Autodesk Inventor part; units mm, degrees
(part 3 of 7)
  arc A519 (-46.3463, -31.4916) -> (-46.3463, -35.4916) centre (-46.3463, -33.4916) ccw
  arc A520 (-46.3463, -31.4916) -> (-46.3463, -35.4916) centre (-46.3463, -33.4916) ccw
  arc A521 (-46.3463, -31.4916) -> (-46.3463, -35.4916) centre (-46.3463, -33.4916) ccw
  arc A522 (-46.3463, -31.4916) -> (-46.3463, -35.4916) centre (-46.3463, -33.4916) ccw
  arc A523 (-46.3463, -31.4916) -> (-46.3463, -35.4916) centre (-46.3463, -33.4916) ccw
  arc A524 (-52.9119, -35.4916) -> (-52.9119, -31.4916) centre (-52.9119, -33.4916) ccw
  arc A525 (-52.9119, -35.4916) -> (-52.9119, -31.4916) centre (-52.9119, -33.4916) ccw
  arc A526 (-52.9119, -35.4916) -> (-52.9119, -31.4916) centre (-52.9119, -33.4916) ccw
  arc A527 (-52.9119, -35.4916) -> (-52.9119, -31.4916) centre (-52.9119, -33.4916) ccw
  line L460 (-42.4124, -24.5346) -> (-55.8468, -24.5346)
  line L461 (-55.8468, -28.5346) -> (-42.4124, -28.5346)
  line L462 (-55.8468, -28.5346) -> (-42.4124, -28.5346)
  line L463 (-55.8468, -28.5346) -> (-42.4124, -28.5346)
  line L464 (-55.8468, -28.5346) -> (-42.4124, -28.5346)
  line L465 (-55.8468, -28.5346) -> (-42.4124, -28.5346)
  line L466 (-42.4124, -24.5346) -> (-55.8468, -24.5346)
  line L467 (-42.4124, -24.5346) -> (-55.8468, -24.5346)
  line L468 (-42.4124, -24.5346) -> (-55.8468, -24.5346)
  line L469 (-42.4124, -24.5346) -> (-55.8468, -24.5346)
  arc A528 (-86.3463, -31.4916) -> (-86.3463, -35.4916) centre (-86.3463, -33.4916) ccw
  arc A529 (-86.3463, -31.4916) -> (-86.3463, -35.4916) centre (-86.3463, -33.4916) ccw
  arc A530 (-86.3463, -31.4916) -> (-86.3463, -35.4916) centre (-86.3463, -33.4916) ccw
  arc A531 (-92.9119, -35.4916) -> (-92.9119, -31.4916) centre (-92.9119, -33.4916) ccw
  line L470 (-82.4124, -24.5346) -> (-95.8468, -24.5346)
  line L471 (-95.8468, -28.5346) -> (-82.4124, -28.5346)
  line L472 (-86.3463, -35.4916) -> (-72.9119, -35.4916)
  line L473 (-86.3463, -35.4916) -> (-72.9119, -35.4916)
  line L474 (-86.3463, -35.4916) -> (-72.9119, -35.4916)
  line L475 (-72.9119, -31.4916) -> (-86.3463, -31.4916)
  line L476 (-72.9119, -31.4916) -> (-86.3463, -31.4916)
  line L477 (-72.9119, -31.4916) -> (-86.3463, -31.4916)
  arc A532 (-75.8468, -24.5346) -> (-75.8468, -28.5346) centre (-75.8468, -26.5346) ccw
  arc A533 (-75.8468, -24.5346) -> (-75.8468, -28.5346) centre (-75.8468, -26.5346) ccw
  arc A534 (-75.8468, -24.5346) -> (-75.8468, -28.5346) centre (-75.8468, -26.5346) ccw
  arc A535 (-75.8468, -24.5346) -> (-75.8468, -28.5346) centre (-75.8468, -26.5346) ccw
  arc A536 (-82.4124, -28.5346) -> (-82.4124, -24.5346) centre (-82.4124, -26.5346) ccw
  line L478 (-66.3463, -35.4916) -> (-52.9119, -35.4916)
  line L479 (-52.9119, -31.4916) -> (-66.3463, -31.4916)
  line L480 (-52.9119, -31.4916) -> (-66.3463, -31.4916)
  line L481 (-66.3463, -35.4916) -> (-52.9119, -35.4916)
  line L482 (-52.9119, -31.4916) -> (-66.3463, -31.4916)
  line L483 (-52.9119, -31.4916) -> (-66.3463, -31.4916)
  line L484 (-52.9119, -31.4916) -> (-66.3463, -31.4916)
  line L485 (-66.3463, -35.4916) -> (-52.9119, -35.4916)
  line L486 (-66.3463, -35.4916) -> (-52.9119, -35.4916)
  line L487 (-66.3463, -35.4916) -> (-52.9119, -35.4916)
  line L488 (-46.3463, -35.4916) -> (-32.9119, -35.4916)
  line L489 (-32.9119, -31.4916) -> (-46.3463, -31.4916)
  line L490 (-32.9119, -31.4916) -> (-46.3463, -31.4916)
  line L491 (-46.3463, -35.4916) -> (-32.9119, -35.4916)
  line L492 (-32.9119, -31.4916) -> (-46.3463, -31.4916)
  line L493 (-32.9119, -31.4916) -> (-46.3463, -31.4916)
  line L494 (-32.9119, -31.4916) -> (-46.3463, -31.4916)
  line L495 (-46.3463, -35.4916) -> (-32.9119, -35.4916)
  line L496 (-46.3463, -35.4916) -> (-32.9119, -35.4916)
  line L497 (-46.3463, -35.4916) -> (-32.9119, -35.4916)
  line L498 (-46.3463, -35.4916) -> (-32.9119, -35.4916)
  line L499 (-32.9119, -31.4916) -> (-46.3463, -31.4916)
  arc A537 (-55.8468, -24.5346) -> (-55.8468, -28.5346) centre (-55.8468, -26.5346) ccw
  arc A538 (-55.8468, -24.5346) -> (-55.8468, -28.5346) centre (-55.8468, -26.5346) ccw
  arc A539 (-55.8468, -24.5346) -> (-55.8468, -28.5346) centre (-55.8468, -26.5346) ccw
  arc A540 (-62.4124, -28.5346) -> (-62.4124, -24.5346) centre (-62.4124, -26.5346) ccw
  arc A541 (-55.8468, -24.5346) -> (-55.8468, -28.5346) centre (-55.8468, -26.5346) ccw
  arc A542 (-55.8468, -24.5346) -> (-55.8468, -28.5346) centre (-55.8468, -26.5346) ccw
  arc A543 (-55.8468, -24.5346) -> (-55.8468, -28.5346) centre (-55.8468, -26.5346) ccw
  arc A544 (-55.8468, -24.5346) -> (-55.8468, -28.5346) centre (-55.8468, -26.5346) ccw
  arc A545 (-62.4124, -28.5346) -> (-62.4124, -24.5346) centre (-62.4124, -26.5346) ccw
  arc A546 (-62.4124, -28.5346) -> (-62.4124, -24.5346) centre (-62.4124, -26.5346) ccw
  arc A547 (-66.3463, -31.4916) -> (-66.3463, -35.4916) centre (-66.3463, -33.4916) ccw
  arc A548 (-72.9119, -35.4916) -> (-72.9119, -31.4916) centre (-72.9119, -33.4916) ccw
  arc A549 (-66.3463, -31.4916) -> (-66.3463, -35.4916) centre (-66.3463, -33.4916) ccw
  line L500 (-62.4124, -24.5346) -> (-75.8468, -24.5346)
  line L501 (-75.8468, -28.5346) -> (-62.4124, -28.5346)
  arc A550 (-72.9119, -35.4916) -> (-72.9119, -31.4916) centre (-72.9119, -33.4916) ccw
  line L502 (-62.4124, -24.5346) -> (-75.8468, -24.5346)
  line L503 (-75.8468, -28.5346) -> (-62.4124, -28.5346)
  arc A551 (-66.3463, -31.4916) -> (-66.3463, -35.4916) centre (-66.3463, -33.4916) ccw
  arc A552 (-66.3463, -31.4916) -> (-66.3463, -35.4916) centre (-66.3463, -33.4916) ccw
  arc A553 (-66.3463, -31.4916) -> (-66.3463, -35.4916) centre (-66.3463, -33.4916) ccw
  line L504 (-62.4124, -24.5346) -> (-75.8468, -24.5346)
  line L505 (-75.8468, -28.5346) -> (-62.4124, -28.5346)
  arc A554 (-72.9119, -35.4916) -> (-72.9119, -31.4916) centre (-72.9119, -33.4916) ccw
  arc A555 (-106.3463, -31.4916) -> (-106.3463, -35.4916) centre (-106.3463, -33.4916) ccw
  arc A556 (-95.8468, -24.5346) -> (-95.8468, -28.5346) centre (-95.8468, -26.5346) ccw
  line L506 (-92.9119, -31.4916) -> (-106.3463, -31.4916)
  line L507 (-106.3463, -35.4916) -> (-92.9119, -35.4916)
  arc A557 (-35.8468, -24.5346) -> (-35.8468, -28.5346) centre (-35.8468, -26.5346) ccw
  arc A558 (-35.8468, -24.5346) -> (-35.8468, -28.5346) centre (-35.8468, -26.5346) ccw
  arc A559 (-35.8468, -24.5346) -> (-35.8468, -28.5346) centre (-35.8468, -26.5346) ccw
  arc A560 (-42.4124, -28.5346) -> (-42.4124, -24.5346) centre (-42.4124, -26.5346) ccw
  arc A561 (-42.4124, -28.5346) -> (-42.4124, -24.5346) centre (-42.4124, -26.5346) ccw
  arc A562 (-35.8468, -24.5346) -> (-35.8468, -28.5346) centre (-35.8468, -26.5346) ccw
  arc A563 (-35.8468, -24.5346) -> (-35.8468, -28.5346) centre (-35.8468, -26.5346) ccw
  arc A564 (-35.8468, -24.5346) -> (-35.8468, -28.5346) centre (-35.8468, -26.5346) ccw
  arc A565 (-35.8468, -24.5346) -> (-35.8468, -28.5346) centre (-35.8468, -26.5346) ccw
  arc A566 (-35.8468, -24.5346) -> (-35.8468, -28.5346) centre (-35.8468, -26.5346) ccw
  arc A567 (-35.8468, -24.5346) -> (-35.8468, -28.5346) centre (-35.8468, -26.5346) ccw
  arc A568 (-42.4124, -28.5346) -> (-42.4124, -24.5346) centre (-42.4124, -26.5346) ccw
  arc A569 (-42.4124, -28.5346) -> (-42.4124, -24.5346) centre (-42.4124, -26.5346) ccw
  arc A570 (-42.4124, -28.5346) -> (-42.4124, -24.5346) centre (-42.4124, -26.5346) ccw
  arc A571 (44.1532, -10.5346) -> (44.1532, -14.5346) centre (44.1532, -12.5346) ccw
  arc A572 (44.1532, -10.5346) -> (44.1532, -14.5346) centre (44.1532, -12.5346) ccw
  arc A573 (44.1532, -10.5346) -> (44.1532, -14.5346) centre (44.1532, -12.5346) ccw
  arc A574 (44.1532, -10.5346) -> (44.1532, -14.5346) centre (44.1532, -12.5346) ccw
  arc A575 (44.1532, -10.5346) -> (44.1532, -14.5346) centre (44.1532, -12.5346) ccw
  arc A576 (44.1532, -10.5346) -> (44.1532, -14.5346) centre (44.1532, -12.5346) ccw
  arc A577 (44.1532, -10.5346) -> (44.1532, -14.5346) centre (44.1532, -12.5346) ccw
  arc A578 (33.6537, -17.4916) -> (33.6537, -21.4916) centre (33.6537, -19.4916) ccw
  arc A579 (27.0881, -21.4916) -> (27.0881, -17.4916) centre (27.0881, -19.4916) ccw
  arc A580 (27.0881, -21.4916) -> (27.0881, -17.4916) centre (27.0881, -19.4916) ccw
  arc A581 (33.6537, -17.4916) -> (33.6537, -21.4916) centre (33.6537, -19.4916) ccw
  arc A582 (27.0881, -21.4916) -> (27.0881, -17.4916) centre (27.0881, -19.4916) ccw
  arc A583 (27.0881, -21.4916) -> (27.0881, -17.4916) centre (27.0881, -19.4916) ccw
  arc A584 (27.0881, -21.4916) -> (27.0881, -17.4916) centre (27.0881, -19.4916) ccw
  arc A585 (27.0881, -21.4916) -> (27.0881, -17.4916) centre (27.0881, -19.4916) ccw
  arc A586 (33.6537, -17.4916) -> (33.6537, -21.4916) centre (33.6537, -19.4916) ccw
  arc A587 (33.6537, -17.4916) -> (33.6537, -21.4916) centre (33.6537, -19.4916) ccw
  arc A588 (33.6537, -17.4916) -> (33.6537, -21.4916) centre (33.6537, -19.4916) ccw
  line L508 (24.1532, -14.5346) -> (37.5876, -14.5346)
  line L509 (37.5876, -10.5346) -> (24.1532, -10.5346)
  line L510 (24.1532, -14.5346) -> (37.5876, -14.5346)
  line L511 (24.1532, -14.5346) -> (37.5876, -14.5346)
  line L512 (24.1532, -14.5346) -> (37.5876, -14.5346)
  line L513 (24.1532, -14.5346) -> (37.5876, -14.5346)
  line L514 (24.1532, -14.5346) -> (37.5876, -14.5346)
  line L515 (37.5876, -10.5346) -> (24.1532, -10.5346)
  line L516 (37.5876, -10.5346) -> (24.1532, -10.5346)
  line L517 (37.5876, -10.5346) -> (24.1532, -10.5346)
  line L518 (37.5876, -10.5346) -> (24.1532, -10.5346)
  line L519 (37.5876, -10.5346) -> (24.1532, -10.5346)
  arc A589 (37.5876, -14.5346) -> (37.5876, -10.5346) centre (37.5876, -12.5346) ccw
  arc A590 (37.5876, -14.5346) -> (37.5876, -10.5346) centre (37.5876, -12.5346) ccw
  arc A591 (37.5876, -14.5346) -> (37.5876, -10.5346) centre (37.5876, -12.5346) ccw
  arc A592 (37.5876, -14.5346) -> (37.5876, -10.5346) centre (37.5876, -12.5346) ccw
  arc A593 (37.5876, -14.5346) -> (37.5876, -10.5346) centre (37.5876, -12.5346) ccw
  arc A594 (37.5876, -14.5346) -> (37.5876, -10.5346) centre (37.5876, -12.5346) ccw
  arc A595 (44.1532, -10.5346) -> (44.1532, -14.5346) centre (44.1532, -12.5346) ccw
  arc A596 (47.0881, -21.4916) -> (47.0881, -17.4916) centre (47.0881, -19.4916) ccw
  arc A597 (47.0881, -21.4916) -> (47.0881, -17.4916) centre (47.0881, -19.4916) ccw
  arc A598 (53.6537, -17.4916) -> (53.6537, -21.4916) centre (53.6537, -19.4916) ccw
  arc A599 (47.0881, -21.4916) -> (47.0881, -17.4916) centre (47.0881, -19.4916) ccw
  arc A600 (47.0881, -21.4916) -> (47.0881, -17.4916) centre (47.0881, -19.4916) ccw
  arc A601 (47.0881, -21.4916) -> (47.0881, -17.4916) centre (47.0881, -19.4916) ccw
  arc A602 (53.6537, -17.4916) -> (53.6537, -21.4916) centre (53.6537, -19.4916) ccw
  arc A603 (53.6537, -17.4916) -> (53.6537, -21.4916) centre (53.6537, -19.4916) ccw
  line L520 (57.5876, -10.5346) -> (44.1532, -10.5346)
  line L521 (44.1532, -14.5346) -> (57.5876, -14.5346)
  line L522 (57.5876, -10.5346) -> (44.1532, -10.5346)
  line L523 (44.1532, -14.5346) -> (57.5876, -14.5346)
  line L524 (44.1532, -14.5346) -> (57.5876, -14.5346)
  line L525 (44.1532, -14.5346) -> (57.5876, -14.5346)
  line L526 (44.1532, -14.5346) -> (57.5876, -14.5346)
  line L527 (57.5876, -10.5346) -> (44.1532, -10.5346)
  line L528 (57.5876, -10.5346) -> (44.1532, -10.5346)
  line L529 (57.5876, -10.5346) -> (44.1532, -10.5346)
  arc A604 (57.5876, -14.5346) -> (57.5876, -10.5346) centre (57.5876, -12.5346) ccw
  arc A605 (64.1532, -10.5346) -> (64.1532, -14.5346) centre (64.1532, -12.5346) ccw
  line L530 (53.6537, -21.4916) -> (67.0881, -21.4916)
  line L531 (53.6537, -21.4916) -> (67.0881, -21.4916)
  line L532 (53.6537, -21.4916) -> (67.0881, -21.4916)
  line L533 (67.0881, -17.4916) -> (53.6537, -17.4916)
  line L534 (67.0881, -17.4916) -> (53.6537, -17.4916)
  line L535 (67.0881, -17.4916) -> (53.6537, -17.4916)
  arc A606 (64.1532, -10.5346) -> (64.1532, -14.5346) centre (64.1532, -12.5346) ccw
  arc A607 (64.1532, -10.5346) -> (64.1532, -14.5346) centre (64.1532, -12.5346) ccw
  arc A608 (64.1532, -10.5346) -> (64.1532, -14.5346) centre (64.1532, -12.5346) ccw
  arc A609 (64.1532, -10.5346) -> (64.1532, -14.5346) centre (64.1532, -12.5346) ccw
  arc A610 (57.5876, -14.5346) -> (57.5876, -10.5346) centre (57.5876, -12.5346) ccw
  arc A611 (57.5876, -14.5346) -> (57.5876, -10.5346) centre (57.5876, -12.5346) ccw
  arc A612 (57.5876, -14.5346) -> (57.5876, -10.5346) centre (57.5876, -12.5346) ccw
  arc A613 (57.5876, -14.5346) -> (57.5876, -10.5346) centre (57.5876, -12.5346) ccw
  arc A614 (67.0881, -21.4916) -> (67.0881, -17.4916) centre (67.0881, -19.4916) ccw
  arc A615 (67.0881, -21.4916) -> (67.0881, -17.4916) centre (67.0881, -19.4916) ccw
  arc A616 (67.0881, -21.4916) -> (67.0881, -17.4916) centre (67.0881, -19.4916) ccw
  line L536 (77.5876, -10.5346) -> (64.1532, -10.5346)
  line L537 (77.5876, -10.5346) -> (64.1532, -10.5346)
  line L538 (77.5876, -10.5346) -> (64.1532, -10.5346)
  line L539 (64.1532, -14.5346) -> (77.5876, -14.5346)
  line L540 (64.1532, -14.5346) -> (77.5876, -14.5346)
  line L541 (64.1532, -14.5346) -> (77.5876, -14.5346)
  arc A617 (73.6537, -17.4916) -> (73.6537, -21.4916) centre (73.6537, -19.4916) ccw
  arc A618 (77.5876, -14.5346) -> (77.5876, -10.5346) centre (77.5876, -12.5346) ccw
  arc A619 (77.5876, -14.5346) -> (77.5876, -10.5346) centre (77.5876, -12.5346) ccw
  arc A620 (77.5876, -14.5346) -> (77.5876, -10.5346) centre (77.5876, -12.5346) ccw
  arc A621 (84.1532, -10.5346) -> (84.1532, -14.5346) centre (84.1532, -12.5346) ccw
  arc A622 (84.1532, -10.5346) -> (84.1532, -14.5346) centre (84.1532, -12.5346) ccw
  line L542 (87.0881, -17.4916) -> (73.6537, -17.4916)
  arc A623 (87.0881, -21.4916) -> (87.0881, -17.4916) centre (87.0881, -19.4916) ccw
  line L543 (73.6537, -21.4916) -> (87.0881, -21.4916)
  line L544 (84.1532, -14.5346) -> (97.5876, -14.5346)
  line L545 (97.5876, -10.5346) -> (84.1532, -10.5346)
  arc A624 (97.5876, -14.5346) -> (97.5876, -10.5346) centre (97.5876, -12.5346) ccw
  line L546 (33.6537, -21.4916) -> (47.0881, -21.4916)
  line L547 (47.0881, -17.4916) -> (33.6537, -17.4916)
  line L548 (33.6537, -21.4916) -> (47.0881, -21.4916)
  line L549 (47.0881, -17.4916) -> (33.6537, -17.4916)
  line L550 (47.0881, -17.4916) -> (33.6537, -17.4916)
  line L551 (47.0881, -17.4916) -> (33.6537, -17.4916)
  line L552 (47.0881, -17.4916) -> (33.6537, -17.4916)
  line L553 (33.6537, -21.4916) -> (47.0881, -21.4916)
  line L554 (33.6537, -21.4916) -> (47.0881, -21.4916)
  line L555 (33.6537, -21.4916) -> (47.0881, -21.4916)
  arc A625 (13.6537, -17.4916) -> (13.6537, -21.4916) centre (13.6537, -19.4916) ccw
  arc A626 (13.6537, -17.4916) -> (13.6537, -21.4916) centre (13.6537, -19.4916) ccw
  arc A627 (13.6537, -17.4916) -> (13.6537, -21.4916) centre (13.6537, -19.4916) ccw
  arc A628 (13.6537, -17.4916) -> (13.6537, -21.4916) centre (13.6537, -19.4916) ccw
  arc A629 (13.6537, -17.4916) -> (13.6537, -21.4916) centre (13.6537, -19.4916) ccw
  arc A630 (13.6537, -17.4916) -> (13.6537, -21.4916) centre (13.6537, -19.4916) ccw
  arc A631 (7.0881, -21.4916) -> (7.0881, -17.4916) centre (7.0881, -19.4916) ccw
  arc A632 (7.0881, -21.4916) -> (7.0881, -17.4916) centre (7.0881, -19.4916) ccw
  arc A633 (7.0881, -21.4916) -> (7.0881, -17.4916) centre (7.0881, -19.4916) ccw
  arc A634 (7.0881, -21.4916) -> (7.0881, -17.4916) centre (7.0881, -19.4916) ccw
  arc A635 (17.5876, -14.5346) -> (17.5876, -10.5346) centre (17.5876, -12.5346) ccw
  arc A636 (17.5876, -14.5346) -> (17.5876, -10.5346) centre (17.5876, -12.5346) ccw
  arc A637 (17.5876, -14.5346) -> (17.5876, -10.5346) centre (17.5876, -12.5346) ccw
  arc A638 (17.5876, -14.5346) -> (17.5876, -10.5346) centre (17.5876, -12.5346) ccw
  arc A639 (17.5876, -14.5346) -> (17.5876, -10.5346) centre (17.5876, -12.5346) ccw
  arc A640 (17.5876, -14.5346) -> (17.5876, -10.5346) centre (17.5876, -12.5346) ccw
  arc A641 (24.1532, -10.5346) -> (24.1532, -14.5346) centre (24.1532, -12.5346) ccw
  arc A642 (24.1532, -10.5346) -> (24.1532, -14.5346) centre (24.1532, -12.5346) ccw
  arc A643 (24.1532, -10.5346) -> (24.1532, -14.5346) centre (24.1532, -12.5346) ccw
  arc A644 (24.1532, -10.5346) -> (24.1532, -14.5346) centre (24.1532, -12.5346) ccw
  arc A645 (24.1532, -10.5346) -> (24.1532, -14.5346) centre (24.1532, -12.5346) ccw
  arc A646 (24.1532, -10.5346) -> (24.1532, -14.5346) centre (24.1532, -12.5346) ccw
  arc A647 (24.1532, -10.5346) -> (24.1532, -14.5346) centre (24.1532, -12.5346) ccw
  arc A648 (24.1532, -10.5346) -> (24.1532, -14.5346) centre (24.1532, -12.5346) ccw
  arc A649 (24.1532, -10.5346) -> (24.1532, -14.5346) centre (24.1532, -12.5346) ccw
  arc A650 (4.1532, -10.5346) -> (4.1532, -14.5346) centre (4.1532, -12.5346) ccw
  arc A651 (4.1532, -10.5346) -> (4.1532, -14.5346) centre (4.1532, -12.5346) ccw
  arc A652 (4.1532, -10.5346) -> (4.1532, -14.5346) centre (4.1532, -12.5346) ccw
  arc A653 (4.1532, -10.5346) -> (4.1532, -14.5346) centre (4.1532, -12.5346) ccw
  arc A654 (4.1532, -10.5346) -> (4.1532, -14.5346) centre (4.1532, -12.5346) ccw
  arc A655 (4.1532, -10.5346) -> (4.1532, -14.5346) centre (4.1532, -12.5346) ccw
  arc A656 (4.1532, -10.5346) -> (4.1532, -14.5346) centre (4.1532, -12.5346) ccw
  arc A657 (4.1532, -10.5346) -> (4.1532, -14.5346) centre (4.1532, -12.5346) ccw
  arc A658 (4.1532, -10.5346) -> (4.1532, -14.5346) centre (4.1532, -12.5346) ccw
  arc A659 (-2.4124, -14.5346) -> (-2.4124, -10.5346) centre (-2.4124, -12.5346) ccw
  arc A660 (-2.4124, -14.5346) -> (-2.4124, -10.5346) centre (-2.4124, -12.5346) ccw
  arc A661 (-2.4124, -14.5346) -> (-2.4124, -10.5346) centre (-2.4124, -12.5346) ccw
  arc A662 (-2.4124, -14.5346) -> (-2.4124, -10.5346) centre (-2.4124, -12.5346) ccw
  arc A663 (-32.9119, -21.4916) -> (-32.9119, -17.4916) centre (-32.9119, -19.4916) ccw
  arc A664 (-32.9119, -21.4916) -> (-32.9119, -17.4916) centre (-32.9119, -19.4916) ccw
  arc A665 (-32.9119, -21.4916) -> (-32.9119, -17.4916) centre (-32.9119, -19.4916) ccw
  arc A666 (-32.9119, -21.4916) -> (-32.9119, -17.4916) centre (-32.9119, -19.4916) ccw
  arc A667 (-32.9119, -21.4916) -> (-32.9119, -17.4916) centre (-32.9119, -19.4916) ccw
  arc A668 (-32.9119, -21.4916) -> (-32.9119, -17.4916) centre (-32.9119, -19.4916) ccw
  line L556 (27.0881, -17.4916) -> (13.6537, -17.4916)
  line L557 (13.6537, -21.4916) -> (27.0881, -21.4916)
  line L558 (27.0881, -17.4916) -> (13.6537, -17.4916)
  line L559 (13.6537, -21.4916) -> (27.0881, -21.4916)
  line L560 (13.6537, -21.4916) -> (27.0881, -21.4916)
  line L561 (27.0881, -17.4916) -> (13.6537, -17.4916)
  line L562 (27.0881, -17.4916) -> (13.6537, -17.4916)
  line L563 (27.0881, -17.4916) -> (13.6537, -17.4916)
  line L564 (13.6537, -21.4916) -> (27.0881, -21.4916)
  line L565 (13.6537, -21.4916) -> (27.0881, -21.4916)
  line L566 (13.6537, -21.4916) -> (27.0881, -21.4916)
  line L567 (27.0881, -17.4916) -> (13.6537, -17.4916)
  line L568 (4.1532, -14.5346) -> (17.5876, -14.5346)
  line L569 (4.1532, -14.5346) -> (17.5876, -14.5346)
  line L570 (4.1532, -14.5346) -> (17.5876, -14.5346)
  line L571 (4.1532, -14.5346) -> (17.5876, -14.5346)
  line L572 (4.1532, -14.5346) -> (17.5876, -14.5346)
  line L573 (4.1532, -14.5346) -> (17.5876, -14.5346)
  line L574 (17.5876, -10.5346) -> (4.1532, -10.5346)
  line L575 (17.5876, -10.5346) -> (4.1532, -10.5346)
  line L576 (17.5876, -10.5346) -> (4.1532, -10.5346)
  line L577 (17.5876, -10.5346) -> (4.1532, -10.5346)
  line L578 (17.5876, -10.5346) -> (4.1532, -10.5346)
  line L579 (17.5876, -10.5346) -> (4.1532, -10.5346)
  arc A669 (7.0881, -21.4916) -> (7.0881, -17.4916) centre (7.0881, -19.4916) ccw
  arc A670 (7.0881, -21.4916) -> (7.0881, -17.4916) centre (7.0881, -19.4916) ccw
  line L580 (-6.3463, -21.4916) -> (7.0881, -21.4916)
  line L581 (7.0881, -17.4916) -> (-6.3463, -17.4916)
  line L582 (7.0881, -17.4916) -> (-6.3463, -17.4916)
  line L583 (-6.3463, -21.4916) -> (7.0881, -21.4916)
  line L584 (-6.3463, -21.4916) -> (7.0881, -21.4916)
  line L585 (7.0881, -17.4916) -> (-6.3463, -17.4916)
  line L586 (7.0881, -17.4916) -> (-6.3463, -17.4916)
  line L587 (7.0881, -17.4916) -> (-6.3463, -17.4916)
  line L588 (-6.3463, -21.4916) -> (7.0881, -21.4916)
  line L589 (-6.3463, -21.4916) -> (7.0881, -21.4916)
  line L590 (-6.3463, -21.4916) -> (7.0881, -21.4916)
  line L591 (7.0881, -17.4916) -> (-6.3463, -17.4916)
  arc A671 (-6.3463, -17.4916) -> (-6.3463, -21.4916) centre (-6.3463, -19.4916) ccw
  arc A672 (-6.3463, -17.4916) -> (-6.3463, -21.4916) centre (-6.3463, -19.4916) ccw
  arc A673 (-6.3463, -17.4916) -> (-6.3463, -21.4916) centre (-6.3463, -19.4916) ccw
  arc A674 (-6.3463, -17.4916) -> (-6.3463, -21.4916) centre (-6.3463, -19.4916) ccw
  arc A675 (-6.3463, -17.4916) -> (-6.3463, -21.4916) centre (-6.3463, -19.4916) ccw
  arc A676 (-6.3463, -17.4916) -> (-6.3463, -21.4916) centre (-6.3463, -19.4916) ccw
  arc A677 (-12.9119, -21.4916) -> (-12.9119, -17.4916) centre (-12.9119, -19.4916) ccw
  arc A678 (-12.9119, -21.4916) -> (-12.9119, -17.4916) centre (-12.9119, -19.4916) ccw
  arc A679 (-12.9119, -21.4916) -> (-12.9119, -17.4916) centre (-12.9119, -19.4916) ccw
  arc A680 (-12.9119, -21.4916) -> (-12.9119, -17.4916) centre (-12.9119, -19.4916) ccw
  arc A681 (-12.9119, -21.4916) -> (-12.9119, -17.4916) centre (-12.9119, -19.4916) ccw
  line L592 (-2.4124, -10.5346) -> (-15.8468, -10.5346)
  line L593 (-15.8468, -14.5346) -> (-2.4124, -14.5346)
  line L594 (-2.4124, -10.5346) -> (-15.8468, -10.5346)
  line L595 (-15.8468, -14.5346) -> (-2.4124, -14.5346)
  line L596 (-2.4124, -10.5346) -> (-15.8468, -10.5346)
  line L597 (-15.8468, -14.5346) -> (-2.4124, -14.5346)
  line L598 (-2.4124, -10.5346) -> (-15.8468, -10.5346)
  line L599 (-15.8468, -14.5346) -> (-2.4124, -14.5346)
  line L600 (-2.4124, -10.5346) -> (-15.8468, -10.5346)
  line L601 (-15.8468, -14.5346) -> (-2.4124, -14.5346)
  line L602 (-15.8468, -14.5346) -> (-2.4124, -14.5346)
  line L603 (-2.4124, -10.5346) -> (-15.8468, -10.5346)
  arc A682 (-2.4124, -14.5346) -> (-2.4124, -10.5346) centre (-2.4124, -12.5346) ccw
  arc A683 (-2.4124, -14.5346) -> (-2.4124, -10.5346) centre (-2.4124, -12.5346) ccw
  arc A684 (-15.8468, -10.5346) -> (-15.8468, -14.5346) centre (-15.8468, -12.5346) ccw
  arc A685 (-15.8468, -10.5346) -> (-15.8468, -14.5346) centre (-15.8468, -12.5346) ccw
  arc A686 (-15.8468, -10.5346) -> (-15.8468, -14.5346) centre (-15.8468, -12.5346) ccw
  arc A687 (-15.8468, -10.5346) -> (-15.8468, -14.5346) centre (-15.8468, -12.5346) ccw
  arc A688 (-15.8468, -10.5346) -> (-15.8468, -14.5346) centre (-15.8468, -12.5346) ccw
  arc A689 (-22.4124, -14.5346) -> (-22.4124, -10.5346) centre (-22.4124, -12.5346) ccw
  arc A690 (-22.4124, -14.5346) -> (-22.4124, -10.5346) centre (-22.4124, -12.5346) ccw
  arc A691 (-15.8468, -10.5346) -> (-15.8468, -14.5346) centre (-15.8468, -12.5346) ccw
  arc A692 (-15.8468, -10.5346) -> (-15.8468, -14.5346) centre (-15.8468, -12.5346) ccw
  arc A693 (-22.4124, -14.5346) -> (-22.4124, -10.5346) centre (-22.4124, -12.5346) ccw
  arc A694 (-15.8468, -10.5346) -> (-15.8468, -14.5346) centre (-15.8468, -12.5346) ccw
  arc A695 (-15.8468, -10.5346) -> (-15.8468, -14.5346) centre (-15.8468, -12.5346) ccw
  arc A696 (-22.4124, -14.5346) -> (-22.4124, -10.5346) centre (-22.4124, -12.5346) ccw
  arc A697 (-22.4124, -14.5346) -> (-22.4124, -10.5346) centre (-22.4124, -12.5346) ccw
  arc A698 (-22.4124, -14.5346) -> (-22.4124, -10.5346) centre (-22.4124, -12.5346) ccw
  arc A699 (-26.3463, -17.4916) -> (-26.3463, -21.4916) centre (-26.3463, -19.4916) ccw
  arc A700 (-26.3463, -17.4916) -> (-26.3463, -21.4916) centre (-26.3463, -19.4916) ccw
  arc A701 (-26.3463, -17.4916) -> (-26.3463, -21.4916) centre (-26.3463, -19.4916) ccw
  arc A702 (-26.3463, -17.4916) -> (-26.3463, -21.4916) centre (-26.3463, -19.4916) ccw
  arc A703 (-26.3463, -17.4916) -> (-26.3463, -21.4916) centre (-26.3463, -19.4916) ccw
  arc A704 (-26.3463, -17.4916) -> (-26.3463, -21.4916) centre (-26.3463, -19.4916) ccw
  line L604 (-35.8468, -14.5346) -> (-22.4124, -14.5346)
  line L605 (-35.8468, -14.5346) -> (-22.4124, -14.5346)
  line L606 (-35.8468, -14.5346) -> (-22.4124, -14.5346)
  line L607 (-35.8468, -14.5346) -> (-22.4124, -14.5346)
  line L608 (-35.8468, -14.5346) -> (-22.4124, -14.5346)
  line L609 (-35.8468, -14.5346) -> (-22.4124, -14.5346)
  line L610 (-22.4124, -10.5346) -> (-35.8468, -10.5346)
  line L611 (-22.4124, -10.5346) -> (-35.8468, -10.5346)
  line L612 (-22.4124, -10.5346) -> (-35.8468, -10.5346)
  line L613 (-22.4124, -10.5346) -> (-35.8468, -10.5346)
  line L614 (-22.4124, -10.5346) -> (-35.8468, -10.5346)
  line L615 (-22.4124, -10.5346) -> (-35.8468, -10.5346)
  line L616 (-26.3463, -21.4916) -> (-12.9119, -21.4916)
  line L617 (-12.9119, -17.4916) -> (-26.3463, -17.4916)
  line L618 (-12.9119, -17.4916) -> (-26.3463, -17.4916)
  line L619 (-26.3463, -21.4916) -> (-12.9119, -21.4916)
  line L620 (-12.9119, -17.4916) -> (-26.3463, -17.4916)
  line L621 (-12.9119, -17.4916) -> (-26.3463, -17.4916)
  line L622 (-26.3463, -21.4916) -> (-12.9119, -21.4916)
  line L623 (-12.9119, -17.4916) -> (-26.3463, -17.4916)
  line L624 (-12.9119, -17.4916) -> (-26.3463, -17.4916)
  line L625 (-26.3463, -21.4916) -> (-12.9119, -21.4916)
  line L626 (-26.3463, -21.4916) -> (-12.9119, -21.4916)
  line L627 (-26.3463, -21.4916) -> (-12.9119, -21.4916)
  arc A705 (-12.9119, -21.4916) -> (-12.9119, -17.4916) centre (-12.9119, -19.4916) ccw
  arc A706 (-46.3463, -17.4916) -> (-46.3463, -21.4916) centre (-46.3463, -19.4916) ccw
  arc A707 (-52.9119, -21.4916) -> (-52.9119, -17.4916) centre (-52.9119, -19.4916) ccw
  arc A708 (-46.3463, -17.4916) -> (-46.3463, -21.4916) centre (-46.3463, -19.4916) ccw
  arc A709 (-46.3463, -17.4916) -> (-46.3463, -21.4916) centre (-46.3463, -19.4916) ccw
  arc A710 (-46.3463, -17.4916) -> (-46.3463, -21.4916) centre (-46.3463, -19.4916) ccw
  arc A711 (-46.3463, -17.4916) -> (-46.3463, -21.4916) centre (-46.3463, -19.4916) ccw
  arc A712 (-46.3463, -17.4916) -> (-46.3463, -21.4916) centre (-46.3463, -19.4916) ccw
  arc A713 (-52.9119, -21.4916) -> (-52.9119, -17.4916) centre (-52.9119, -19.4916) ccw
  arc A714 (-52.9119, -21.4916) -> (-52.9119, -17.4916) centre (-52.9119, -19.4916) ccw
  arc A715 (-52.9119, -21.4916) -> (-52.9119, -17.4916) centre (-52.9119, -19.4916) ccw
  arc A716 (-52.9119, -21.4916) -> (-52.9119, -17.4916) centre (-52.9119, -19.4916) ccw
  line L628 (-42.4124, -10.5346) -> (-55.8468, -10.5346)
  line L629 (-55.8468, -14.5346) -> (-42.4124, -14.5346)
  line L630 (-55.8468, -14.5346) -> (-42.4124, -14.5346)
  line L631 (-55.8468, -14.5346) -> (-42.4124, -14.5346)
  line L632 (-55.8468, -14.5346) -> (-42.4124, -14.5346)
  line L633 (-55.8468, -14.5346) -> (-42.4124, -14.5346)
  line L634 (-42.4124, -10.5346) -> (-55.8468, -10.5346)
  line L635 (-42.4124, -10.5346) -> (-55.8468, -10.5346)
  line L636 (-42.4124, -10.5346) -> (-55.8468, -10.5346)
  line L637 (-42.4124, -10.5346) -> (-55.8468, -10.5346)
  arc A717 (-86.3463, -17.4916) -> (-86.3463, -21.4916) centre (-86.3463, -19.4916) ccw
  arc A718 (-86.3463, -17.4916) -> (-86.3463, -21.4916) centre (-86.3463, -19.4916) ccw
  arc A719 (-86.3463, -17.4916) -> (-86.3463, -21.4916) centre (-86.3463, -19.4916) ccw
  arc A720 (-92.9119, -21.4916) -> (-92.9119, -17.4916) centre (-92.9119, -19.4916) ccw
  line L638 (-82.4124, -10.5346) -> (-95.8468, -10.5346)
  line L639 (-95.8468, -14.5346) -> (-82.4124, -14.5346)
  line L640 (-86.3463, -21.4916) -> (-72.9119, -21.4916)
  line L641 (-86.3463, -21.4916) -> (-72.9119, -21.4916)
  line L642 (-86.3463, -21.4916) -> (-72.9119, -21.4916)
  line L643 (-72.9119, -17.4916) -> (-86.3463, -17.4916)
  line L644 (-72.9119, -17.4916) -> (-86.3463, -17.4916)
  line L645 (-72.9119, -17.4916) -> (-86.3463, -17.4916)
  arc A721 (-75.8468, -10.5346) -> (-75.8468, -14.5346) centre (-75.8468, -12.5346) ccw
  arc A722 (-75.8468, -10.5346) -> (-75.8468, -14.5346) centre (-75.8468, -12.5346) ccw
  arc A723 (-75.8468, -10.5346) -> (-75.8468, -14.5346) centre (-75.8468, -12.5346) ccw
  arc A724 (-75.8468, -10.5346) -> (-75.8468, -14.5346) centre (-75.8468, -12.5346) ccw
  arc A725 (-82.4124, -14.5346) -> (-82.4124, -10.5346) centre (-82.4124, -12.5346) ccw
  line L646 (-66.3463, -21.4916) -> (-52.9119, -21.4916)
  line L647 (-52.9119, -17.4916) -> (-66.3463, -17.4916)
  line L648 (-52.9119, -17.4916) -> (-66.3463, -17.4916)
  line L649 (-66.3463, -21.4916) -> (-52.9119, -21.4916)
  line L650 (-52.9119, -17.4916) -> (-66.3463, -17.4916)
  line L651 (-52.9119, -17.4916) -> (-66.3463, -17.4916)
  line L652 (-52.9119, -17.4916) -> (-66.3463, -17.4916)
  line L653 (-66.3463, -21.4916) -> (-52.9119, -21.4916)
  line L654 (-66.3463, -21.4916) -> (-52.9119, -21.4916)
  line L655 (-66.3463, -21.4916) -> (-52.9119, -21.4916)
  line L656 (-46.3463, -21.4916) -> (-32.9119, -21.4916)
  line L657 (-32.9119, -17.4916) -> (-46.3463, -17.4916)
  line L658 (-32.9119, -17.4916) -> (-46.3463, -17.4916)
  line L659 (-46.3463, -21.4916) -> (-32.9119, -21.4916)
  line L660 (-32.9119, -17.4916) -> (-46.3463, -17.4916)
  line L661 (-32.9119, -17.4916) -> (-46.3463, -17.4916)
  line L662 (-32.9119, -17.4916) -> (-46.3463, -17.4916)
  line L663 (-46.3463, -21.4916) -> (-32.9119, -21.4916)
  line L664 (-46.3463, -21.4916) -> (-32.9119, -21.4916)
  line L665 (-46.3463, -21.4916) -> (-32.9119, -21.4916)
  line L666 (-46.3463, -21.4916) -> (-32.9119, -21.4916)
  line L667 (-32.9119, -17.4916) -> (-46.3463, -17.4916)
  arc A726 (-55.8468, -10.5346) -> (-55.8468, -14.5346) centre (-55.8468, -12.5346) ccw
  arc A727 (-55.8468, -10.5346) -> (-55.8468, -14.5346) centre (-55.8468, -12.5346) ccw
  arc A728 (-55.8468, -10.5346) -> (-55.8468, -14.5346) centre (-55.8468, -12.5346) ccw
  arc A729 (-62.4124, -14.5346) -> (-62.4124, -10.5346) centre (-62.4124, -12.5346) ccw
  arc A730 (-55.8468, -10.5346) -> (-55.8468, -14.5346) centre (-55.8468, -12.5346) ccw
  arc A731 (-55.8468, -10.5346) -> (-55.8468, -14.5346) centre (-55.8468, -12.5346) ccw
  arc A732 (-55.8468, -10.5346) -> (-55.8468, -14.5346) centre (-55.8468, -12.5346) ccw
  arc A733 (-55.8468, -10.5346) -> (-55.8468, -14.5346) centre (-55.8468, -12.5346) ccw
  arc A734 (-62.4124, -14.5346) -> (-62.4124, -10.5346) centre (-62.4124, -12.5346) ccw
  arc A735 (-62.4124, -14.5346) -> (-62.4124, -10.5346) centre (-62.4124, -12.5346) ccw
  arc A736 (-66.3463, -17.4916) -> (-66.3463, -21.4916) centre (-66.3463, -19.4916) ccw
  arc A737 (-72.9119, -21.4916) -> (-72.9119, -17.4916) centre (-72.9119, -19.4916) ccw
  arc A738 (-66.3463, -17.4916) -> (-66.3463, -21.4916) centre (-66.3463, -19.4916) ccw
  line L668 (-62.4124, -10.5346) -> (-75.8468, -10.5346)
  line L669 (-75.8468, -14.5346) -> (-62.4124, -14.5346)
  arc A739 (-72.9119, -21.4916) -> (-72.9119, -17.4916) centre (-72.9119, -19.4916) ccw
  line L670 (-62.4124, -10.5346) -> (-75.8468, -10.5346)
  line L671 (-75.8468, -14.5346) -> (-62.4124, -14.5346)
  arc A740 (-66.3463, -17.4916) -> (-66.3463, -21.4916) centre (-66.3463, -19.4916) ccw
  arc A741 (-66.3463, -17.4916) -> (-66.3463, -21.4916) centre (-66.3463, -19.4916) ccw
  arc A742 (-66.3463, -17.4916) -> (-66.3463, -21.4916) centre (-66.3463, -19.4916) ccw
  line L672 (-62.4124, -10.5346) -> (-75.8468, -10.5346)
  line L673 (-75.8468, -14.5346) -> (-62.4124, -14.5346)
  arc A743 (-72.9119, -21.4916) -> (-72.9119, -17.4916) centre (-72.9119, -19.4916) ccw
  arc A744 (-106.3463, -17.4916) -> (-106.3463, -21.4916) centre (-106.3463, -19.4916) ccw
  arc A745 (-95.8468, -10.5346) -> (-95.8468, -14.5346) centre (-95.8468, -12.5346) ccw
  line L674 (-92.9119, -17.4916) -> (-106.3463, -17.4916)
  line L675 (-106.3463, -21.4916) -> (-92.9119, -21.4916)
  arc A746 (-35.8468, -10.5346) -> (-35.8468, -14.5346) centre (-35.8468, -12.5346) ccw
  arc A747 (-35.8468, -10.5346) -> (-35.8468, -14.5346) centre (-35.8468, -12.5346) ccw
  arc A748 (-35.8468, -10.5346) -> (-35.8468, -14.5346) centre (-35.8468, -12.5346) ccw
  arc A749 (-42.4124, -14.5346) -> (-42.4124, -10.5346) centre (-42.4124, -12.5346) ccw
  arc A750 (-42.4124, -14.5346) -> (-42.4124, -10.5346) centre (-42.4124, -12.5346) ccw
  arc A751 (-35.8468, -10.5346) -> (-35.8468, -14.5346) centre (-35.8468, -12.5346) ccw
  arc A752 (-35.8468, -10.5346) -> (-35.8468, -14.5346) centre (-35.8468, -12.5346) ccw
  arc A753 (-35.8468, -10.5346) -> (-35.8468, -14.5346) centre (-35.8468, -12.5346) ccw
  arc A754 (-35.8468, -10.5346) -> (-35.8468, -14.5346) centre (-35.8468, -12.5346) ccw
  arc A755 (-35.8468, -10.5346) -> (-35.8468, -14.5346) centre (-35.8468, -12.5346) ccw
  arc A756 (-35.8468, -10.5346) -> (-35.8468, -14.5346) centre (-35.8468, -12.5346) ccw
  arc A757 (-42.4124, -14.5346) -> (-42.4124, -10.5346) centre (-42.4124, -12.5346) ccw
  arc A758 (-42.4124, -14.5346) -> (-42.4124, -10.5346) centre (-42.4124, -12.5346) ccw
  arc A759 (-42.4124, -14.5346) -> (-42.4124, -10.5346) centre (-42.4124, -12.5346) ccw
  arc A760 (44.1532, 3.4654) -> (44.1532, -0.5346) centre (44.1532, 1.4654) ccw
  arc A761 (44.1532, 3.4654) -> (44.1532, -0.5346) centre (44.1532, 1.4654) ccw
  arc A762 (44.1532, 3.4654) -> (44.1532, -0.5346) centre (44.1532, 1.4654) ccw
  arc A763 (44.1532, 3.4654) -> (44.1532, -0.5346) centre (44.1532, 1.4654) ccw
  arc A764 (44.1532, 3.4654) -> (44.1532, -0.5346) centre (44.1532, 1.4654) ccw
  arc A765 (44.1532, 3.4654) -> (44.1532, -0.5346) centre (44.1532, 1.4654) ccw
  arc A766 (44.1532, 3.4654) -> (44.1532, -0.5346) centre (44.1532, 1.4654) ccw
  arc A767 (33.6537, -3.4916) -> (33.6537, -7.4916) centre (33.6537, -5.4916) ccw
  arc A768 (27.0881, -7.4916) -> (27.0881, -3.4916) centre (27.0881, -5.4916) ccw
  arc A769 (27.0881, -7.4916) -> (27.0881, -3.4916) centre (27.0881, -5.4916) ccw
  arc A770 (33.6537, -3.4916) -> (33.6537, -7.4916) centre (33.6537, -5.4916) ccw
  arc A771 (27.0881, -7.4916) -> (27.0881, -3.4916) centre (27.0881, -5.4916) ccw
  arc A772 (27.0881, -7.4916) -> (27.0881, -3.4916) centre (27.0881, -5.4916) ccw
  arc A773 (27.0881, -7.4916) -> (27.0881, -3.4916) centre (27.0881, -5.4916) ccw
  arc A774 (27.0881, -7.4916) -> (27.0881, -3.4916) centre (27.0881, -5.4916) ccw
  arc A775 (33.6537, -3.4916) -> (33.6537, -7.4916) centre (33.6537, -5.4916) ccw
  arc A776 (33.6537, -3.4916) -> (33.6537, -7.4916) centre (33.6537, -5.4916) ccw
  arc A777 (33.6537, -3.4916) -> (33.6537, -7.4916) centre (33.6537, -5.4916) ccw
  line L676 (24.1532, -0.5346) -> (37.5876, -0.5346)
  line L677 (37.5876, 3.4654) -> (24.1532, 3.4654)
  line L678 (24.1532, -0.5346) -> (37.5876, -0.5346)
  line L679 (24.1532, -0.5346) -> (37.5876, -0.5346)
  line L680 (24.1532, -0.5346) -> (37.5876, -0.5346)
  line L681 (24.1532, -0.5346) -> (37.5876, -0.5346)
  line L682 (24.1532, -0.5346) -> (37.5876, -0.5346)
  line L683 (37.5876, 3.4654) -> (24.1532, 3.4654)
  line L684 (37.5876, 3.4654) -> (24.1532, 3.4654)
  line L685 (37.5876, 3.4654) -> (24.1532, 3.4654)
  line L686 (37.5876, 3.4654) -> (24.1532, 3.4654)
  line L687 (37.5876, 3.4654) -> (24.1532, 3.4654)
  arc A778 (37.5876, -0.5346) -> (37.5876, 3.4654) centre (37.5876, 1.4654) ccw
  arc A779 (37.5876, -0.5346) -> (37.5876, 3.4654) centre (37.5876, 1.4654) ccw
  arc A780 (37.5876, -0.5346) -> (37.5876, 3.4654) centre (37.5876, 1.4654) ccw
  arc A781 (37.5876, -0.5346) -> (37.5876, 3.4654) centre (37.5876, 1.4654) ccw
  arc A782 (37.5876, -0.5346) -> (37.5876, 3.4654) centre (37.5876, 1.4654) ccw
  arc A783 (37.5876, -0.5346) -> (37.5876, 3.4654) centre (37.5876, 1.4654) ccw
  arc A784 (44.1532, 3.4654) -> (44.1532, -0.5346) centre (44.1532, 1.4654) ccw
  arc A785 (47.0881, -7.4916) -> (47.0881, -3.4916) centre (47.0881, -5.4916) ccw
  arc A786 (47.0881, -7.4916) -> (47.0881, -3.4916) centre (47.0881, -5.4916) ccw
  arc A787 (53.6537, -3.4916) -> (53.6537, -7.4916) centre (53.6537, -5.4916) ccw
  arc A788 (47.0881, -7.4916) -> (47.0881, -3.4916) centre (47.0881, -5.4916) ccw
  arc A789 (47.0881, -7.4916) -> (47.0881, -3.4916) centre (47.0881, -5.4916) ccw
  arc A790 (47.0881, -7.4916) -> (47.0881, -3.4916) centre (47.0881, -5.4916) ccw
  arc A791 (53.6537, -3.4916) -> (53.6537, -7.4916) centre (53.6537, -5.4916) ccw
  arc A792 (53.6537, -3.4916) -> (53.6537, -7.4916) centre (53.6537, -5.4916) ccw
  line L688 (57.5876, 3.4654) -> (44.1532, 3.4654)
  line L689 (44.1532, -0.5346) -> (57.5876, -0.5346)
  line L690 (57.5876, 3.4654) -> (44.1532, 3.4654)
  line L691 (44.1532, -0.5346) -> (57.5876, -0.5346)
  line L692 (44.1532, -0.5346) -> (57.5876, -0.5346)
  line L693 (44.1532, -0.5346) -> (57.5876, -0.5346)
  line L694 (44.1532, -0.5346) -> (57.5876, -0.5346)
  line L695 (57.5876, 3.4654) -> (44.1532, 3.4654)
  line L696 (57.5876, 3.4654) -> (44.1532, 3.4654)
  line L697 (57.5876, 3.4654) -> (44.1532, 3.4654)
  arc A793 (57.5876, -0.5346) -> (57.5876, 3.4654) centre (57.5876, 1.4654) ccw
  arc A794 (64.1532, 3.4654) -> (64.1532, -0.5346) centre (64.1532, 1.4654) ccw
  line L698 (53.6537, -7.4916) -> (67.0881, -7.4916)
  line L699 (53.6537, -7.4916) -> (67.0881, -7.4916)
  line L700 (53.6537, -7.4916) -> (67.0881, -7.4916)
  line L701 (67.0881, -3.4916) -> (53.6537, -3.4916)
  line L702 (67.0881, -3.4916) -> (53.6537, -3.4916)
  line L703 (67.0881, -3.4916) -> (53.6537, -3.4916)
  arc A795 (64.1532, 3.4654) -> (64.1532, -0.5346) centre (64.1532, 1.4654) ccw
  arc A796 (64.1532, 3.4654) -> (64.1532, -0.5346) centre (64.1532, 1.4654) ccw
  arc A797 (64.1532, 3.4654) -> (64.1532, -0.5346) centre (64.1532, 1.4654) ccw
  arc A798 (64.1532, 3.4654) -> (64.1532, -0.5346) centre (64.1532, 1.4654) ccw
  arc A799 (57.5876, -0.5346) -> (57.5876, 3.4654) centre (57.5876, 1.4654) ccw
  arc A800 (57.5876, -0.5346) -> (57.5876, 3.4654) centre (57.5876, 1.4654) ccw
  arc A801 (57.5876, -0.5346) -> (57.5876, 3.4654) centre (57.5876, 1.4654) ccw
  arc A802 (57.5876, -0.5346) -> (57.5876, 3.4654) centre (57.5876, 1.4654) ccw
  arc A803 (67.0881, -7.4916) -> (67.0881, -3.4916) centre (67.0881, -5.4916) ccw
  arc A804 (67.0881, -7.4916) -> (67.0881, -3.4916) centre (67.0881, -5.4916) ccw
  arc A805 (67.0881, -7.4916) -> (67.0881, -3.4916) centre (67.0881, -5.4916) ccw
  line L704 (77.5876, 3.4654) -> (64.1532, 3.4654)
  line L705 (77.5876, 3.4654) -> (64.1532, 3.4654)
  line L706 (77.5876, 3.4654) -> (64.1532, 3.4654)
  line L707 (64.1532, -0.5346) -> (77.5876, -0.5346)
  line L708 (64.1532, -0.5346) -> (77.5876, -0.5346)
  line L709 (64.1532, -0.5346) -> (77.5876, -0.5346)
  arc A806 (73.6537, -3.4916) -> (73.6537, -7.4916) centre (73.6537, -5.4916) ccw
  arc A807 (77.5876, -0.5346) -> (77.5876, 3.4654) centre (77.5876, 1.4654) ccw
  arc A808 (77.5876, -0.5346) -> (77.5876, 3.4654) centre (77.5876, 1.4654) ccw
  arc A809 (77.5876, -0.5346) -> (77.5876, 3.4654) centre (77.5876, 1.4654) ccw
  arc A810 (84.1532, 3.4654) -> (84.1532, -0.5346) centre (84.1532, 1.4654) ccw
  arc A811 (84.1532, 3.4654) -> (84.1532, -0.5346) centre (84.1532, 1.4654) ccw
  line L710 (87.0881, -3.4916) -> (73.6537, -3.4916)
  arc A812 (87.0881, -7.4916) -> (87.0881, -3.4916) centre (87.0881, -5.4916) ccw
  line L711 (73.6537, -7.4916) -> (87.0881, -7.4916)
  line L712 (84.1532, -0.5346) -> (97.5876, -0.5346)
  line L713 (97.5876, 3.4654) -> (84.1532, 3.4654)
  arc A813 (97.5876, -0.5346) -> (97.5876, 3.4654) centre (97.5876, 1.4654) ccw
  line L714 (33.6537, -7.4916) -> (47.0881, -7.4916)
  line L715 (47.0881, -3.4916) -> (33.6537, -3.4916)
  line L716 (33.6537, -7.4916) -> (47.0881, -7.4916)
  line L717 (47.0881, -3.4916) -> (33.6537, -3.4916)
  line L718 (47.0881, -3.4916) -> (33.6537, -3.4916)
  line L719 (47.0881, -3.4916) -> (33.6537, -3.4916)
  line L720 (47.0881, -3.4916) -> (33.6537, -3.4916)
  line L721 (33.6537, -7.4916) -> (47.0881, -7.4916)
  line L722 (33.6537, -7.4916) -> (47.0881, -7.4916)
  line L723 (33.6537, -7.4916) -> (47.0881, -7.4916)
  arc A814 (13.6537, -3.4916) -> (13.6537, -7.4916) centre (13.6537, -5.4916) ccw
  arc A815 (13.6537, -3.4916) -> (13.6537, -7.4916) centre (13.6537, -5.4916) ccw
  arc A816 (13.6537, -3.4916) -> (13.6537, -7.4916) centre (13.6537, -5.4916) ccw
  arc A817 (13.6537, -3.4916) -> (13.6537, -7.4916) centre (13.6537, -5.4916) ccw
  arc A818 (13.6537, -3.4916) -> (13.6537, -7.4916) centre (13.6537, -5.4916) ccw
  arc A819 (13.6537, -3.4916) -> (13.6537, -7.4916) centre (13.6537, -5.4916) ccw
  arc A820 (7.0881, -7.4916) -> (7.0881, -3.4916) centre (7.0881, -5.4916) ccw
  arc A821 (7.0881, -7.4916) -> (7.0881, -3.4916) centre (7.0881, -5.4916) ccw
  arc A822 (7.0881, -7.4916) -> (7.0881, -3.4916) centre (7.0881, -5.4916) ccw
  arc A823 (7.0881, -7.4916) -> (7.0881, -3.4916) centre (7.0881, -5.4916) ccw
  arc A824 (17.5876, -0.5346) -> (17.5876, 3.4654) centre (17.5876, 1.4654) ccw
  arc A825 (17.5876, -0.5346) -> (17.5876, 3.4654) centre (17.5876, 1.4654) ccw
  arc A826 (17.5876, -0.5346) -> (17.5876, 3.4654) centre (17.5876, 1.4654) ccw
  arc A827 (17.5876, -0.5346) -> (17.5876, 3.4654) centre (17.5876, 1.4654) ccw
  arc A828 (17.5876, -0.5346) -> (17.5876, 3.4654) centre (17.5876, 1.4654) ccw
  arc A829 (17.5876, -0.5346) -> (17.5876, 3.4654) centre (17.5876, 1.4654) ccw
  arc A830 (24.1532, 3.4654) -> (24.1532, -0.5346) centre (24.1532, 1.4654) ccw
  arc A831 (24.1532, 3.4654) -> (24.1532, -0.5346) centre (24.1532, 1.4654) ccw
  arc A832 (24.1532, 3.4654) -> (24.1532, -0.5346) centre (24.1532, 1.4654) ccw
  arc A833 (24.1532, 3.4654) -> (24.1532, -0.5346) centre (24.1532, 1.4654) ccw
  arc A834 (24.1532, 3.4654) -> (24.1532, -0.5346) centre (24.1532, 1.4654) ccw
  arc A835 (24.1532, 3.4654) -> (24.1532, -0.5346) centre (24.1532, 1.4654) ccw
  arc A836 (24.1532, 3.4654) -> (24.1532, -0.5346) centre (24.1532, 1.4654) ccw
  arc A837 (24.1532, 3.4654) -> (24.1532, -0.5346) centre (24.1532, 1.4654) ccw
  arc A838 (24.1532, 3.4654) -> (24.1532, -0.5346) centre (24.1532, 1.4654) ccw
  arc A839 (4.1532, 3.4654) -> (4.1532, -0.5346) centre (4.1532, 1.4654) ccw
  arc A840 (4.1532, 3.4654) -> (4.1532, -0.5346) centre (4.1532, 1.4654) ccw
  arc A841 (4.1532, 3.4654) -> (4.1532, -0.5346) centre (4.1532, 1.4654) ccw
  arc A842 (4.1532, 3.4654) -> (4.1532, -0.5346) centre (4.1532, 1.4654) ccw
  arc A843 (4.1532, 3.4654) -> (4.1532, -0.5346) centre (4.1532, 1.4654) ccw
  arc A844 (4.1532, 3.4654) -> (4.1532, -0.5346) centre (4.1532, 1.4654) ccw
  arc A845 (4.1532, 3.4654) -> (4.1532, -0.5346) centre (4.1532, 1.4654) ccw
  arc A846 (4.1532, 3.4654) -> (4.1532, -0.5346) centre (4.1532, 1.4654) ccw
  arc A847 (4.1532, 3.4654) -> (4.1532, -0.5346) centre (4.1532, 1.4654) ccw
  arc A848 (-2.4124, -0.5346) -> (-2.4124, 3.4654) centre (-2.4124, 1.4654) ccw
  arc A849 (-2.4124, -0.5346) -> (-2.4124, 3.4654) centre (-2.4124, 1.4654) ccw
  arc A850 (-2.4124, -0.5346) -> (-2.4124, 3.4654) centre (-2.4124, 1.4654) ccw
  arc A851 (-2.4124, -0.5346) -> (-2.4124, 3.4654) centre (-2.4124, 1.4654) ccw
  arc A852 (-32.9119, -7.4916) -> (-32.9119, -3.4916) centre (-32.9119, -5.4916) ccw
  arc A853 (-32.9119, -7.4916) -> (-32.9119, -3.4916) centre (-32.9119, -5.4916) ccw
  arc A854 (-32.9119, -7.4916) -> (-32.9119, -3.4916) centre (-32.9119, -5.4916) ccw
  arc A855 (-32.9119, -7.4916) -> (-32.9119, -3.4916) centre (-32.9119, -5.4916) ccw
  arc A856 (-32.9119, -7.4916) -> (-32.9119, -3.4916) centre (-32.9119, -5.4916) ccw
  arc A857 (-32.9119, -7.4916) -> (-32.9119, -3.4916) centre (-32.9119, -5.4916) ccw
  line L724 (27.0881, -3.4916) -> (13.6537, -3.4916)
  line L725 (13.6537, -7.4916) -> (27.0881, -7.4916)
  line L726 (27.0881, -3.4916) -> (13.6537, -3.4916)
  line L727 (13.6537, -7.4916) -> (27.0881, -7.4916)
  line L728 (13.6537, -7.4916) -> (27.0881, -7.4916)
  line L729 (27.0881, -3.4916) -> (13.6537, -3.4916)
  line L730 (27.0881, -3.4916) -> (13.6537, -3.4916)
  line L731 (27.0881, -3.4916) -> (13.6537, -3.4916)
  line L732 (13.6537, -7.4916) -> (27.0881, -7.4916)
  line L733 (13.6537, -7.4916) -> (27.0881, -7.4916)
  line L734 (13.6537, -7.4916) -> (27.0881, -7.4916)
  line L735 (27.0881, -3.4916) -> (13.6537, -3.4916)
  line L736 (4.1532, -0.5346) -> (17.5876, -0.5346)
  line L737 (4.1532, -0.5346) -> (17.5876, -0.5346)
  line L738 (4.1532, -0.5346) -> (17.5876, -0.5346)
  line L739 (4.1532, -0.5346) -> (17.5876, -0.5346)
  line L740 (4.1532, -0.5346) -> (17.5876, -0.5346)
  line L741 (4.1532, -0.5346) -> (17.5876, -0.5346)
  line L742 (17.5876, 3.4654) -> (4.1532, 3.4654)
  line L743 (17.5876, 3.4654) -> (4.1532, 3.4654)
  line L744 (17.5876, 3.4654) -> (4.1532, 3.4654)
  line L745 (17.5876, 3.4654) -> (4.1532, 3.4654)
  line L746 (17.5876, 3.4654) -> (4.1532, 3.4654)
  line L747 (17.5876, 3.4654) -> (4.1532, 3.4654)
  arc A858 (7.0881, -7.4916) -> (7.0881, -3.4916) centre (7.0881, -5.4916) ccw
  arc A859 (7.0881, -7.4916) -> (7.0881, -3.4916) centre (7.0881, -5.4916) ccw
  line L748 (-6.3463, -7.4916) -> (7.0881, -7.4916)
  line L749 (7.0881, -3.4916) -> (-6.3463, -3.4916)
  line L750 (7.0881, -3.4916) -> (-6.3463, -3.4916)
  line L751 (-6.3463, -7.4916) -> (7.0881, -7.4916)
  line L752 (-6.3463, -7.4916) -> (7.0881, -7.4916)
  line L753 (7.0881, -3.4916) -> (-6.3463, -3.4916)
  line L754 (7.0881, -3.4916) -> (-6.3463, -3.4916)
  line L755 (7.0881, -3.4916) -> (-6.3463, -3.4916)
  line L756 (-6.3463, -7.4916) -> (7.0881, -7.4916)
  line L757 (-6.3463, -7.4916) -> (7.0881, -7.4916)
  line L758 (-6.3463, -7.4916) -> (7.0881, -7.4916)
  line L759 (7.0881, -3.4916) -> (-6.3463, -3.4916)
  arc A860 (-6.3463, -3.4916) -> (-6.3463, -7.4916) centre (-6.3463, -5.4916) ccw
  arc A861 (-6.3463, -3.4916) -> (-6.3463, -7.4916) centre (-6.3463, -5.4916) ccw
  arc A862 (-6.3463, -3.4916) -> (-6.3463, -7.4916) centre (-6.3463, -5.4916) ccw
  arc A863 (-6.3463, -3.4916) -> (-6.3463, -7.4916) centre (-6.3463, -5.4916) ccw
  arc A864 (-6.3463, -3.4916) -> (-6.3463, -7.4916) centre (-6.3463, -5.4916) ccw
  arc A865 (-6.3463, -3.4916) -> (-6.3463, -7.4916) centre (-6.3463, -5.4916) ccw
  arc A866 (-12.9119, -7.4916) -> (-12.9119, -3.4916) centre (-12.9119, -5.4916) ccw
  arc A867 (-12.9119, -7.4916) -> (-12.9119, -3.4916) centre (-12.9119, -5.4916) ccw
  arc A868 (-12.9119, -7.4916) -> (-12.9119, -3.4916) centre (-12.9119, -5.4916) ccw
  arc A869 (-12.9119, -7.4916) -> (-12.9119, -3.4916) centre (-12.9119, -5.4916) ccw
  arc A870 (-12.9119, -7.4916) -> (-12.9119, -3.4916) centre (-12.9119, -5.4916) ccw
  line L760 (-2.4124, 3.4654) -> (-15.8468, 3.4654)
  line L761 (-15.8468, -0.5346) -> (-2.4124, -0.5346)
  line L762 (-2.4124, 3.4654) -> (-15.8468, 3.4654)
  line L763 (-15.8468, -0.5346) -> (-2.4124, -0.5346)
  line L764 (-2.4124, 3.4654) -> (-15.8468, 3.4654)
  line L765 (-15.8468, -0.5346) -> (-2.4124, -0.5346)
  line L766 (-2.4124, 3.4654) -> (-15.8468, 3.4654)
  line L767 (-15.8468, -0.5346) -> (-2.4124, -0.5346)
  line L768 (-2.4124, 3.4654) -> (-15.8468, 3.4654)
  line L769 (-15.8468, -0.5346) -> (-2.4124, -0.5346)
  line L770 (-15.8468, -0.5346) -> (-2.4124, -0.5346)
  line L771 (-2.4124, 3.4654) -> (-15.8468, 3.4654)
  arc A871 (-2.4124, -0.5346) -> (-2.4124, 3.4654) centre (-2.4124, 1.4654) ccw
  arc A872 (-2.4124, -0.5346) -> (-2.4124, 3.4654) centre (-2.4124, 1.4654) ccw
  arc A873 (-15.8468, 3.4654) -> (-15.8468, -0.5346) centre (-15.8468, 1.4654) ccw
  arc A874 (-15.8468, 3.4654) -> (-15.8468, -0.5346) centre (-15.8468, 1.4654) ccw
  arc A875 (-15.8468, 3.4654) -> (-15.8468, -0.5346) centre (-15.8468, 1.4654) ccw
  arc A876 (-15.8468, 3.4654) -> (-15.8468, -0.5346) centre (-15.8468, 1.4654) ccw
  arc A877 (-15.8468, 3.4654) -> (-15.8468, -0.5346) centre (-15.8468, 1.4654) ccw
  arc A878 (-22.4124, -0.5346) -> (-22.4124, 3.4654) centre (-22.4124, 1.4654) ccw
  arc A879 (-22.4124, -0.5346) -> (-22.4124, 3.4654) centre (-22.4124, 1.4654) ccw
  arc A880 (-15.8468, 3.4654) -> (-15.8468, -0.5346) centre (-15.8468, 1.4654) ccw
  arc A881 (-15.8468, 3.4654) -> (-15.8468, -0.5346) centre (-15.8468, 1.4654) ccw
  arc A882 (-22.4124, -0.5346) -> (-22.4124, 3.4654) centre (-22.4124, 1.4654) ccw
  arc A883 (-15.8468, 3.4654) -> (-15.8468, -0.5346) centre (-15.8468, 1.4654) ccw
  arc A884 (-15.8468, 3.4654) -> (-15.8468, -0.5346) centre (-15.8468, 1.4654) ccw
  arc A885 (-22.4124, -0.5346) -> (-22.4124, 3.4654) centre (-22.4124, 1.4654) ccw
  arc A886 (-22.4124, -0.5346) -> (-22.4124, 3.4654) centre (-22.4124, 1.4654) ccw
  arc A887 (-22.4124, -0.5346) -> (-22.4124, 3.4654) centre (-22.4124, 1.4654) ccw
  arc A888 (-26.3463, -3.4916) -> (-26.3463, -7.4916) centre (-26.3463, -5.4916) ccw
  arc A889 (-26.3463, -3.4916) -> (-26.3463, -7.4916) centre (-26.3463, -5.4916) ccw
  arc A890 (-26.3463, -3.4916) -> (-26.3463, -7.4916) centre (-26.3463, -5.4916) ccw
  arc A891 (-26.3463, -3.4916) -> (-26.3463, -7.4916) centre (-26.3463, -5.4916) ccw
  arc A892 (-26.3463, -3.4916) -> (-26.3463, -7.4916) centre (-26.3463, -5.4916) ccw
  arc A893 (-26.3463, -3.4916) -> (-26.3463, -7.4916) centre (-26.3463, -5.4916) ccw
  line L772 (-35.8468, -0.5346) -> (-22.4124, -0.5346)
  line L773 (-35.8468, -0.5346) -> (-22.4124, -0.5346)
  line L774 (-35.8468, -0.5346) -> (-22.4124, -0.5346)
  line L775 (-35.8468, -0.5346) -> (-22.4124, -0.5346)
  line L776 (-35.8468, -0.5346) -> (-22.4124, -0.5346)
  line L777 (-35.8468, -0.5346) -> (-22.4124, -0.5346)
  line L778 (-22.4124, 3.4654) -> (-35.8468, 3.4654)
  line L779 (-22.4124, 3.4654) -> (-35.8468, 3.4654)
  line L780 (-22.4124, 3.4654) -> (-35.8468, 3.4654)
  line L781 (-22.4124, 3.4654) -> (-35.8468, 3.4654)
  line L782 (-22.4124, 3.4654) -> (-35.8468, 3.4654)
  line L783 (-22.4124, 3.4654) -> (-35.8468, 3.4654)
  line L784 (-26.3463, -7.4916) -> (-12.9119, -7.4916)
  line L785 (-12.9119, -3.4916) -> (-26.3463, -3.4916)
  line L786 (-12.9119, -3.4916) -> (-26.3463, -3.4916)
  line L787 (-26.3463, -7.4916) -> (-12.9119, -7.4916)
  line L788 (-12.9119, -3.4916) -> (-26.3463, -3.4916)
  line L789 (-12.9119, -3.4916) -> (-26.3463, -3.4916)
  line L790 (-26.3463, -7.4916) -> (-12.9119, -7.4916)